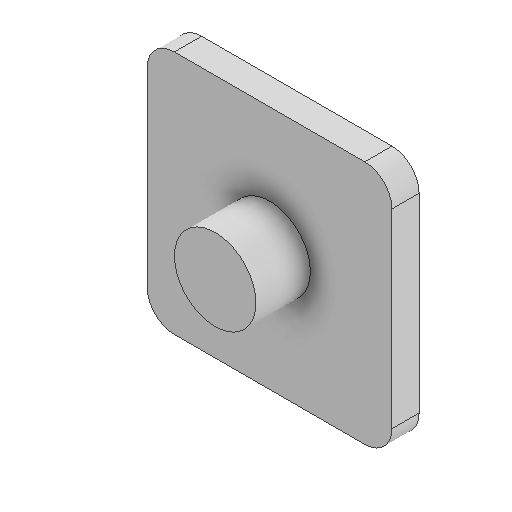
# Autodesk Inventor part: Base
Saved by Autodesk Inventor 2025.2 (Build 292293000, 293)
## iProperties
Created: 2025-03-03
Part Number: Base
Material: Generic
Document SubType Name: Modeling
Designer: Marcu
Density: 1 g/cm^3
Appearance: Default
Author: Marcu
Autodesk Inventor part; units mm, degrees
ref_plane "YZ Plane" through (0, 0, 0) normal (1, 0, 0) x (0, 1, 0)
ref_plane "XZ Plane" through (0, 0, 0) normal (0, 1, 0) x (-1, 0, 0)
ref_plane "XY Plane" through (0, 0, 0) normal (0, 0, 1) x (1, 0, 0)
sketch "Sketch1" plane through (0, 0, 0) normal (0, 1, 0) x (-1, 0, 0)
  line L0 (22.5, 22.5) -> (-22.5, 22.5)
  line L1 (-22.5, 22.5) -> (-22.5, -22.5)
  line L2 (-22.5, -22.5) -> (22.5, -22.5)
  line L3 (22.5, -22.5) -> (22.5, 22.5)
  point P0 (0, 0)
  dimension "d0" = 45
  dimension "d1" = 45
  dimension "d2" = 22.5
  dimension "d3" = 22.5
  constraints: 8 end point, 2 parallel, 1 horizontal, 1 perpendicular
  measures "d0" distance between parallel lines of L2 L0
  measures "d1" distance between parallel lines of L1 L3
  measures "d2" distance from line of point (0, 0) L2
  measures "d3" distance from line of point (0, 0) L1
extrude "Extrusion1" add sketch "Sketch1" along normal blind 5
sketch "Sketch2" plane through (0, 0, 0) normal (0, -1, 0) x (1, 0, 0)
  circle A0 centre (0, 0) radius 7.5
  dimension "d6" = 15
  constraints: 1 centre point, 1 coincident
  measures "d6" diameter of A0
extrude "Extrusion2" add sketch "Sketch2" along normal blind 10
sketch "Sketch3" plane through (0, 5, 0) normal (0, 1, 0) x (1, 0, 0)
  line L0 (-10, -10) -> (10, -10)
  line L1 (10, -10) -> (10, 10)
  line L2 (10, 10) -> (-10, 10)
  line L3 (-10, 10) -> (-10, -10)
  point P0 (0, 0)
  dimension "d9" = 20
  dimension "d10" = 20
  dimension "d11" = 10
  dimension "d12" = 10
  constraints: 8 end point, 2 parallel, 1 horizontal, 1 perpendicular
  measures "d9" distance between parallel lines of L0 L2
  measures "d10" distance between parallel lines of L1 L3
  measures "d11" distance from line of point (0, 0) L0
  measures "d12" distance from line of point (0, 0) L1
extrude "Extrusion3" cut sketch "Sketch3" against normal blind 2
sketch "Sketch4" plane through (0, 5, 0) normal (0, 1, 0) x (1, 0, 0)
  line L0 (-10, -10) -> (-10, 10) projected
  line L1 (-22.5, 22.5) -> (-22.5, -22.5) projected
  circle A0 centre (-16.25, 0) radius 2.5
  line L2 (10, -10) -> (-10, -10) projected
  line L3 (-10, 10) -> (10, 10) projected
  circle A1 centre (16.25, 0) radius 2.5
  point P0 (0, 0)
  dimension "d15" = 5
  constraints: 2 centre point
  measures "d15" diameter of A0
extrude "Extrusion4" cut sketch "Sketch4" against normal blind 3
fillet "Fillet1" radius 5 4 edges at (22.5, 2.5, 22.5) (22.5, 2.5, -22.5) (-22.5, 2.5, -22.5) (-22.5, 2.5, 22.5)
body "Solid1"
